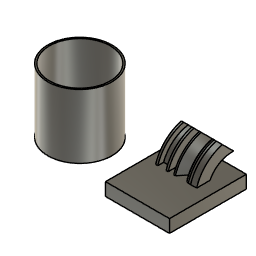
letra (Autodesk Fusion 360 design; units mm, degrees)
Autodesk Fusion 360 part; units mm, degrees
note: some values were not read from the file. Chosen so that the rebuilt part matches the saved one: that a step has no effect.
sketch "Boceto1" plane through (0, 0, 0) normal (0, 0, 1) x (1, 0, 0)
  line L0 (50, 60) -> (-50, 60)
  line L1 (-50, 60) -> (-50, -60)
  line L2 (-50, -60) -> (50, -60)
  line L3 (50, -60) -> (50, 60)
  line L4 (50, 60) -> (-50, -60) construction
  line L5 (-50, 60) -> (50, -60) construction
  dimension "d1" = 100
  dimension "d2" = 120
  constraint horizontal L0
  constraint perpendicular L0 L1
  constraint parallel L0 L2
  constraint parallel L1 L3
  constraint coincident L4 origin
  constraint coincident L5 origin
  measures "d1" distance of L1.end L2.end
  measures "d2" distance of L0.end L1.end
extrude "Extruir1" add sketch "Boceto1" along normal blind 20 makes body 1
ref_plane "PlanoDeObra1" through (0, -60, 20) normal (0, 0.707107, 0.707107) x (1, 0, 0)
ref_plane "PlanoDeObra2" through (0, 10.7107, 90.7107) normal (0, 0.707107, 0.707107) x (1, 0, 0)
sketch "Boceto2" plane through (0, 50.7107, 50.7107) normal (0, 0.707107, 0.707107) x (1, 0, 0)
  line L0 (29.8755, 13.5994) -> (29.8755, -11.4006)
  line L1 (29.8755, -11.4006) -> (20.4451, -11.4006)
  spline S0 degree 2 poles (20.4451, -11.4006) (17.9553, -11.4006) (16.6422, -11.1618) knots 0 0 0 1 1 1
  spline S1 degree 2 poles (16.6422, -11.1618) (14.8004, -10.8549) (13.5556, -9.9937) knots 0 0 0 1 1 1
  spline S2 degree 2 poles (13.5556, -9.9937) (12.3107, -9.1325) (11.5518, -7.5806) knots 0 0 0 1 1 1
  spline S3 degree 2 poles (11.5518, -7.5806) (10.7929, -6.0288) (10.7929, -4.17) knots 0 0 0 1 1 1
  spline S4 degree 2 poles (10.7929, -4.17) (10.7929, -0.9811) (12.8223, 1.2273) knots 0 0 0 1 1 1
  spline S5 degree 2 poles (12.8223, 1.2273) (14.8516, 3.4357) (20.1552, 3.4357) knots 0 0 0 1 1 1
  line L2 (20.1552, 3.4357) -> (26.5672, 3.4357)
  line L3 (26.5672, 3.4357) -> (26.5672, 13.5994)
  line L4 (26.5672, 13.5994) -> (29.8755, 13.5994)
  line L5 (26.5672, 0.4855) -> (20.104, 0.4855)
  spline S6 degree 2 poles (20.104, 0.4855) (16.898, 0.4855) (15.5508, -0.7082) knots 0 0 0 1 1 1
  spline S7 degree 2 poles (15.5508, -0.7082) (14.2036, -1.9019) (14.2036, -4.0677) knots 0 0 0 1 1 1
  spline S8 degree 2 poles (14.2036, -4.0677) (14.2036, -5.6366) (14.9966, -6.7536) knots 0 0 0 1 1 1
  spline S9 degree 2 poles (14.9966, -6.7536) (15.7895, -7.8705) (17.0856, -8.2287) knots 0 0 0 1 1 1
  spline S10 degree 2 poles (17.0856, -8.2287) (17.9212, -8.4504) (20.1722, -8.4504) knots 0 0 0 1 1 1
  line L6 (20.1722, -8.4504) -> (26.5672, -8.4504)
  line L7 (26.5672, -8.4504) -> (26.5672, 0.4855)
  line L8 (-2.7848, 13.5994) -> (-2.7848, 7.6138)
  line L9 (-2.7848, 7.6138) -> (8.061, 7.6138)
  line L10 (8.061, 7.6138) -> (8.061, 4.8)
  line L11 (8.061, 4.8) -> (-3.3476, -11.4006)
  line L12 (-3.3476, -11.4006) -> (-5.8544, -11.4006)
  line L13 (-5.8544, -11.4006) -> (-5.8544, 4.8)
  line L14 (-5.8544, 4.8) -> (-9.2309, 4.8)
  line L15 (-9.2309, 4.8) -> (-9.2309, 7.6138)
  line L16 (-9.2309, 7.6138) -> (-5.8544, 7.6138)
  line L17 (-5.8544, 7.6138) -> (-5.8544, 13.5994)
  line L18 (-5.8544, 13.5994) -> (-2.7848, 13.5994)
  line L19 (-2.7848, 4.8) -> (-2.7848, -6.4722)
  line L20 (-2.7848, -6.4722) -> (5.0426, 4.8)
  line L21 (5.0426, 4.8) -> (-2.7848, 4.8)
  line L22 (-14.4867, 13.5994) -> (-14.4867, -11.4006)
  line L23 (-14.4867, -11.4006) -> (-17.795, -11.4006)
  line L24 (-17.795, -11.4006) -> (-17.795, -1.1345)
  line L25 (-17.795, -1.1345) -> (-30.7896, -1.1345)
  line L26 (-30.7896, -1.1345) -> (-30.7896, -11.4006)
  line L27 (-30.7896, -11.4006) -> (-34.0979, -11.4006)
  line L28 (-34.0979, -11.4006) -> (-34.0979, 13.5994)
  line L29 (-34.0979, 13.5994) -> (-30.7896, 13.5994)
  line L30 (-30.7896, 13.5994) -> (-30.7896, 1.8157)
  line L31 (-30.7896, 1.8157) -> (-17.795, 1.8157)
  line L32 (-17.795, 1.8157) -> (-17.795, 13.5994)
  line L33 (-17.795, 13.5994) -> (-14.4867, 13.5994)
sketch "Boceto3" plane through (0, 0, 0) normal (1, 0, 0) x (0, 1, 0)
  arc A0 (42.6493, 58.7721) -> (0, 0) centre (57.534, 3.1099) ccw
  point P0 (42.6493, 58.7721)
  constraint coincident A0.end origin
  constraint coincident P0 A0.start
sweep "Barrido1" add profiles "Boceto2" path "Boceto3" along A0 section 1 bodies 1
cylinder "CilindroPrimitivo1" add diameter 100 height 100 placed x (1, 0, 0) y (0, 1, 0) z (0, 0, 1) at (-150, 0, 0) separate body makes body 2
ref_plane "PlanoDeObra3" through (-210, 0, 0) normal (1, 0, 0) x (0, 1, 0)
sketch "Boceto5" plane through (-210, 0, 0) normal (1, 0, 0) x (0, 1, 0)
  line L0 (6.4017, 17.5112) -> (6.393, 22.5112)
  line L1 (6.393, 22.5112) -> (4.5069, 22.5079)
  spline S0 degree 2 poles (4.5069, 22.5079) (4.0089, 22.507) (3.7464, 22.4588) knots 0 0 0 1 1 1
  spline S1 degree 2 poles (3.7464, 22.4588) (3.3781, 22.3968) (3.1295, 22.2241) knots 0 0 0 1 1 1
  spline S2 degree 2 poles (3.1295, 22.2241) (2.8808, 22.0514) (2.7296, 21.7408) knots 0 0 0 1 1 1
  spline S3 degree 2 poles (2.7296, 21.7408) (2.5783, 21.4302) (2.579, 21.0584) knots 0 0 0 1 1 1
  spline S4 degree 2 poles (2.579, 21.0584) (2.5801, 20.4206) (2.9867, 19.9797) knots 0 0 0 1 1 1
  spline S5 degree 2 poles (2.9867, 19.9797) (3.3934, 19.5387) (4.4541, 19.5405) knots 0 0 0 1 1 1
  line L2 (4.4541, 19.5405) -> (5.7365, 19.5428)
  line L3 (5.7365, 19.5428) -> (5.74, 17.5101)
  line L4 (5.74, 17.5101) -> (6.4017, 17.5112)
  line L5 (5.7355, 20.1328) -> (4.4428, 20.1306)
  spline S6 degree 2 poles (4.4428, 20.1306) (3.8016, 20.1294) (3.5318, 20.3677) knots 0 0 0 1 1 1
  spline S7 degree 2 poles (3.5318, 20.3677) (3.2619, 20.606) (3.2611, 21.0391) knots 0 0 0 1 1 1
  spline S8 degree 2 poles (3.2611, 21.0391) (3.2606, 21.3529) (3.4188, 21.5766) knots 0 0 0 1 1 1
  spline S9 degree 2 poles (3.4188, 21.5766) (3.577, 21.8003) (3.8361, 21.8723) knots 0 0 0 1 1 1
  spline S10 degree 2 poles (3.8361, 21.8723) (4.0031, 21.917) (4.4533, 21.9178) knots 0 0 0 1 1 1
  line L6 (4.4533, 21.9178) -> (5.7323, 21.92)
  line L7 (5.7323, 21.92) -> (5.7355, 20.1328)
  line L8 (-0.1303, 17.4998) -> (-0.1324, 18.6969)
  line L9 (-0.1324, 18.6969) -> (2.0367, 18.7007)
  line L10 (2.0367, 18.7007) -> (2.0357, 19.2635)
  line L11 (2.0357, 19.2635) -> (-0.2517, 22.4996)
  line L12 (-0.2517, 22.4996) -> (-0.753, 22.4987)
  line L13 (-0.753, 22.4987) -> (-0.7473, 19.2586)
  line L14 (-0.7473, 19.2586) -> (-1.4226, 19.2574)
  line L15 (-1.4226, 19.2574) -> (-1.4217, 18.6946)
  line L16 (-1.4217, 18.6946) -> (-0.7464, 18.6958)
  line L17 (-0.7464, 18.6958) -> (-0.7443, 17.4987)
  line L18 (-0.7443, 17.4987) -> (-0.1303, 17.4998)
  line L19 (-0.1334, 19.2597) -> (-0.1374, 21.5141)
  line L20 (-0.1374, 21.5141) -> (1.4321, 19.2624)
  line L21 (1.4321, 19.2624) -> (-0.1334, 19.2597)
  line L22 (-2.4707, 17.4957) -> (-2.4795, 22.4957)
  line L23 (-2.4795, 22.4957) -> (-3.1411, 22.4945)
  line L24 (-3.1411, 22.4945) -> (-3.1375, 20.4413)
  line L25 (-3.1375, 20.4413) -> (-5.7364, 20.4367)
  line L26 (-5.7364, 20.4367) -> (-5.74, 22.4899)
  line L27 (-5.74, 22.4899) -> (-6.4017, 22.4888)
  line L28 (-6.4017, 22.4888) -> (-6.3929, 17.4888)
  line L29 (-6.3929, 17.4888) -> (-5.7313, 17.49)
  line L30 (-5.7313, 17.49) -> (-5.7354, 19.8467)
  line L31 (-5.7354, 19.8467) -> (-3.1365, 19.8513)
  line L32 (-3.1365, 19.8513) -> (-3.1324, 17.4945)
  line L33 (-3.1324, 17.4945) -> (-2.4707, 17.4957)
emboss "Repujado1" depth -2 profiles "Boceto5" section 1 onto face at (-100.2485, -4.9784, 66.6667) on bodies 2 bodies 2
sketch "Boceto6" plane through (0, 0, 100) normal (0, 0, 1) x (-1, 0, 0)
  circle A0 centre (150, 0) radius 50
  circle A1 centre (150, 0) radius 47.5
  dimension "d22" = 95
  constraint concentric A0 A1
  measures "d22" diameter of A1
extrude "Extruir2" cut sketch "Boceto6" against normal blind 100 contours A1 bodies 2
move_face "MoveFace1" [no effect]
move_body "Desplazar1" bodies 2 to x (0, -1, 0) y (1, 0, 0) z (0, 0, 1) at (-150, -150, 0)
